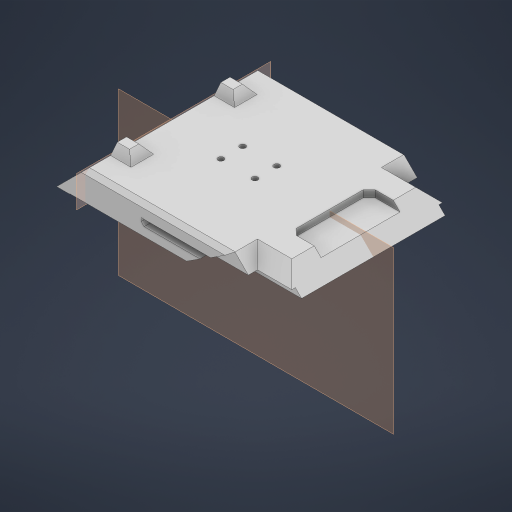
# Autodesk Inventor part: Head_Top
Saved by Autodesk Inventor 2024 (Build 280153000, 153)
## iProperties
Created: 2025-09-25
Part Number: Head_Top
Material: Generic
Document SubType Name: Modeling
Designer: kevin
Density: 1 g/cm^3
Appearance: Default
Author: kevin
Autodesk Inventor part; units mm, degrees
sketch "Sketch1" plane through (0, 0, 0) normal (0, 0, 1) x (1, 0, 0)
  line L0 (-49.5014, 88.2576) -> (-59.1834, 88.2576) projected
  line L1 (-18.2147, 2.3576) -> (-22.3392, 2.3576) projected
  arc A0 (-18.2147, 2.3576) -> (21.128, 5.3576) centre (0, 22.9604) ccw projected
  line L2 (103.9182, 5.3576) -> (21.128, 5.3576) projected
  line L3 (113.8557, 15.2951) -> (103.9182, 5.3576) projected
  line L4 (113.8557, 93.4201) -> (113.8557, 15.2951) projected
  line L5 (103.9182, 103.3576) -> (113.8557, 93.4201) projected
  line L6 (-46.9118, 103.3576) -> (103.9182, 103.3576) projected
  line L7 (-69.3743, 80.8951) -> (-46.9118, 103.3576) projected
  line L8 (-69.3743, 10.0256) -> (-69.3743, 80.8951) projected
  line L9 (-58.7063, -0.6424) -> (-69.3743, 10.0256) projected
  line L10 (-23.5178, -0.6424) -> (-58.7063, -0.6424) projected
  line L11 (-22.3392, 2.3576) -> (-23.5178, -0.6424) projected
  line L12 (-40.6109, 71.1084) -> (-33.5378, 60.1538) projected
  line L13 (-33.5378, 60.1538) -> (-15.7647, 71.6293) projected
  line L14 (-15.7647, 71.6293) -> (-15.7647, 88.2576) projected
  line L15 (-15.7647, 88.2576) -> (35.7434, 88.2576) projected
  line L16 (35.7434, 88.2576) -> (-58.3243, 27.521) projected
  line L17 (-58.3243, 27.521) -> (-58.3243, 44.1499) projected
  line L18 (-58.3243, 44.1499) -> (-49.3014, 49.9757) projected
  line L19 (-49.3014, 49.9757) -> (-49.3014, 71.1084) projected
  line L20 (-49.3014, 71.1084) -> (-40.6109, 71.1084) projected
  line L21 (3.2088, 99.2576) -> (52.78, 99.2576) projected
  line L22 (52.78, 99.2576) -> (46.5848, 95.2576) projected
  line L23 (46.5848, 95.2576) -> (5.2088, 95.2576) projected
  line L24 (3.2088, 97.2576) -> (5.2088, 95.2576) projected
  line L25 (3.2088, 97.2576) -> (3.2088, 99.2576) projected
  circle A1 centre (63.0077, 89.876) radius 2.1 projected
  line L26 (67.5987, 77.171) -> (76.5778, 68.1919) projected
  line L27 (76.5778, 68.1919) -> (76.5778, 21.8886) projected
  line L28 (76.5778, 21.8886) -> (68.2692, 13.58) projected
  line L29 (68.2692, 13.58) -> (19.2393, 13.58) projected
  line L30 (19.2393, 13.58) -> (11.6235, 21.1957) projected
  line L31 (11.6235, 21.1957) -> (67.5987, 77.171) projected
  line L32 (-59.1834, 88.2576) -> (-67.3743, 80.0667) projected
  line L33 (-59.1834, 88.2576) -> (-38.0834, 109.3576)
  line L34 (-46.9118, 103.3576) -> (103.9182, 103.3576) projected
  line L35 (68.9757, 109.3576) -> (117.3307, 109.3576) projected
  line L36 (68.9757, 109.3576) -> (-38.0834, 109.3576)
  line L37 (53.7977, 99.5576) -> (2.9088, 99.5576)
  line L38 (2.9088, 99.5576) -> (2.9088, 97.1333)
  line L39 (2.9088, 97.1333) -> (5.0845, 94.9576)
  line L40 (5.0845, 94.9576) -> (46.6733, 94.9576)
  line L41 (46.6733, 94.9576) -> (53.7977, 99.5576)
  line L42 (36.7611, 88.5576) -> (-16.0647, 88.5576)
  line L43 (-16.0647, 88.5576) -> (-16.0647, 71.7927)
  line L44 (-16.0647, 71.7927) -> (-33.4485, 60.5685)
  line L45 (-33.4485, 60.5685) -> (-40.4475, 71.4084)
  line L46 (-40.4475, 71.4084) -> (-49.6014, 71.4084)
  line L47 (-49.6014, 71.4084) -> (-49.6014, 50.1391)
  line L48 (-49.6014, 50.1391) -> (-58.6243, 44.3133)
  line L49 (-58.6243, 44.3133) -> (-58.6243, 26.9702)
  line L50 (-58.6243, 26.9702) -> (36.7611, 88.5576)
  line L51 (-16.0647, 88.5576) -> (-49.5014, 88.5576)
  line L52 (-49.5014, 88.5576) -> (-49.5014, 88.2576)
  line L53 (-56.6516, 28.2439) -> (64.3294, 106.3576) projected
  line L54 (-56.8143, 28.4959) -> (68.4226, 109.3576)
  line L55 (68.9757, 109.3576) -> (64.3294, 106.3576)
  point P0 (0, 0)
  point P1 (36.208, 88.5576)
  point P2 (46.1202, 94.9576)
  point P3 (53.2446, 99.5576)
  dimension "d0" = 0.3
  dimension "d1" = 0.3
  dimension "d2" = 0.3
  constraints: 40 end point, 2 horizontal, 1 parallel, 1 perpendicular, 1 point on line, 15 other
  measures "d0" distance between parallel lines of L21 L37
  measures "d1" distance between parallel lines of L15 L42
  measures "d2" distance between parallel lines of L53 L54
ref_plane "Work Plane1" through (-15.7647, 88.2576, 9.8) normal (0, 0.7071068, -0.7071068) x (0, 0.7071068, 0.7071068)
extrude "Extrusion1" add sketch "Sketch1" against normal up to surface contours L0 L33 L6 L54 L37 L38 L39 L40 L42 L51 L52 | L33 L36 L54 L6 | L54 L36 L55 L53 L6 | L6 L53 L37 L54 surface through (-15.7647, 88.2576, 9.8) normal (0, 0.7071068, -0.7071068)
ref_plane "Work Plane2" through (0, 0, 64.8) normal (0, 0, 1) x (1, 0, 0)
sketch "Sketch2" plane through (0, 0, 64.8) normal (0, 0, 1) x (1, 0, 0)
  line L0 (119.8557, 83.6682) -> (110.6663, 92.8576) projected
  line L1 (99.1663, 104.3576) -> (94.1663, 109.3576) projected
  line L2 (68.9757, 109.3576) -> (-38.0834, 109.3576) projected
  line L3 (-59.1834, 88.2576) -> (-49.5014, 88.2576) projected
  line L4 (-38.0834, 109.3576) -> (-59.1834, 88.2576) projected
  line L5 (68.9757, 109.3576) -> (94.1663, 109.3576) projected
  line L6 (-56.6516, 28.2439) -> (64.3294, 106.3576) projected
  line L7 (-56.6516, 28.2439) -> (64.3294, 106.3576) projected
  line L8 (53.7977, 99.5576) -> (68.9757, 109.3576) projected
  line L9 (-49.5014, 88.2576) -> (-49.5014, 88.5576) projected
  line L10 (-49.5014, 88.5576) -> (36.208, 88.5576) projected
  line L11 (46.1202, 94.9576) -> (5.0845, 94.9576) projected
  line L12 (46.1202, 94.9576) -> (46.6733, 94.9576)
  line L13 (5.0845, 94.9576) -> (-36.1716, 94.9576)
  line L14 (-36.1716, 94.9576) -> (-42.5716, 88.5576)
  point P0 (0, 0)
  dimension "d5" = 135
  constraints: 6 end point, 3 point on line, 1 horizontal
  measures "d5" angle of L13 L14
extrude "Extrusion2" add sketch "Sketch2" against normal up to surface surface through (4.8962, 98.8076, 20.35) normal (0, 0.7071068, -0.7071068)
sketch "Sketch3" plane through (0, 0, 64.8) normal (0, 0, 1) x (1, 0, 0)
  line L0 (119.8557, 83.6682) -> (110.6663, 92.8576) projected
  line L1 (99.1663, 104.3576) -> (94.1663, 109.3576) projected
  line L2 (68.9757, 109.3576) -> (94.1663, 109.3576) projected
  line L3 (99.1663, 104.3576) -> (112.3307, 104.3576) projected
  line L4 (110.6663, 92.8576) -> (99.1663, 104.3576)
  line L5 (-36.1716, 94.9576) -> (46.6733, 94.9576) projected
  line L6 (46.6733, 94.9576) -> (108.5663, 94.9576)
  line L7 (46.6733, 94.9576) -> (68.9757, 109.3576) projected
  line L8 (68.9757, 109.3576) -> (85.4757, 92.8576) projected
  line L9 (68.9757, 109.3576) -> (83.3757, 94.9576)
  line L10 (108.5663, 94.9576) -> (94.1663, 109.3576)
  line L11 (68.9757, 109.3576) -> (94.1663, 109.3576)
  point P0 (0, 0)
  constraints: 10 end point, 3 point on line, 2 collinear, 1 horizontal
ref_plane "Work Plane3" through (-8.0243, 5.3576, 2.8) normal (0, 0, 1) x (1, 0, 0)
extrude "Extrusion3" add sketch "Sketch3" against normal up to surface (62 mm away) contours L8 L6 L7
sketch "Sketch4" plane through (0, 0, 64.8) normal (0, 0, 1) x (1, 0, 0)
  line L0 (94.1663, 109.3576) -> (110.6663, 92.8576) projected
  line L1 (68.9757, 109.3576) -> (117.3307, 109.3576) projected
  line L2 (68.9757, 109.3576) -> (85.4757, 92.8576) projected
  line L3 (46.6733, 94.9576) -> (108.5663, 94.9576) projected
  point P0 (0, 0)
  point P1 (83.3757, 94.9576)
ref_plane "Work Plane4" through (68.9757, 92.8576, 2.8) normal (0, -0.7071068, 0.7071068) x (1, 0, 0)
extrude "Extrusion4" add sketch "Sketch4" against normal up to surface surface through (68.9757, 92.8576, 2.8) normal (0, -0.7071068, 0.7071068)
ref_plane "Work Plane5" through (7.9088, 97.1333, 0) normal (1, 0, 0) x (0, 0, -1)
sketch "Sketch6" plane through (7.9088, 97.1333, 0) normal (1, 0, 0) x (0, 0, -1)
  line L0 (0, -2.1757) -> (-16.5, -2.1757) projected
  line L1 (0.2, 0.1243) -> (0.2, -1.8757) projected
  line L2 (0.2, 0.1243) -> (0.2, 2.1243) projected
  line L3 (0, 2.4243) -> (-21.1, 2.4243) projected
  line L4 (-16.5, -2.1757) -> (-18.6757, 0) projected
  line L5 (-18.6757, 0) -> (-21.1, 2.4243) projected
  line L6 (0.2, 2.1243) -> (0.2, 2.4243)
  line L7 (0.2, 2.4243) -> (0, 2.4243)
  line L8 (0.2, -1.8757) -> (0, -2.1757)
  line L9 (-11.8, -25.504) -> (-11.8, -6.8757) projected
  line L10 (-12.1, -25.504) -> (-12.1, 2.4243)
  point P0 (0, -97.1333)
  point P1 (-12.1, -2.1757)
  dimension "d13" = 0.3
  constraints: 8 end point, 1 collinear, 1 parallel, 1 point on line, 1 vertical
  measures "d13" distance between parallel lines of L9 L10
extrude "Extrusion5" cut sketch "Sketch6" along normal blind 163.5125 contours L0 L10 L3 L7 L6 L2 L1 L8
chamfer "Chamfer1" distance 3 angle 45 1 edges at (15.4462, 109.3576, 0)
sketch "Sketch8" plane through (0, 0, 64.8) normal (0, 0, 1) x (1, 0, 0)
  line L0 (99.1663, 104.3576) -> (94.1663, 109.3576) projected
  line L1 (94.1663, 109.3576) -> (-38.0834, 109.3576) projected
  line L2 (99.1663, 104.3576) -> (76.5047, 104.3576)
  line L3 (76.5047, 104.3576) -> (71.5047, 109.3576)
  line L4 (108.5663, 94.9576) -> (94.1663, 109.3576) projected
  line L5 (76.5047, 104.3576) -> (76.5047, 109.3576)
  point P0 (0, 0)
  constraints: 6 end point, 2 point on line, 1 horizontal, 1 parallel, 1 perpendicular
ref_plane "Work Plane6" through (94.1663, 34.1725, 35.8) normal (0, 0, 1) x (1, 0, 0)
extrude "Extrusion6" cut sketch "Sketch8" against normal up to surface (29 mm away) contours L2 L5 L1 L0
mirror "Mirror2" about plane through (0, 0, 64.8) normal (0, 0, 1) of "Extrusion1", "Extrusion2", "Extrusion3", "Extrusion4", "Extrusion5", "Chamfer1", "Extrusion6"
sketch "Sketch10" plane through (-49.5014, 88.5576, 0) normal (0, -1, 0) x (1, 0, 0)
  line L0 (0, 129.6) -> (0, 0) projected
  circle A0 centre (5.406, 102.8115) radius 2.1
  circle A1 centre (5.406, 102.8115) radius 4.6
  line L1 (-43.2319, 64.8) -> (191.6177, 64.8) construction
  circle A2 centre (5.406, 102.8115) radius 5.1
  circle A3 centre (5.406, 26.7885) radius 2.1
  circle A4 centre (5.406, 26.7885) radius 4.6
  circle A5 centre (5.406, 26.7885) radius 5.1
  point P0 (49.5014, 0)
  dimension "d23" = 4.2
  dimension "d24" = 2.5
  dimension "d25" = 0.5
  constraints: 6 centre point, 1 symmetric about line, 3 other
  measures "d23" diameter of A0
  measures "d24" radial gap between concentric circles of A0 A1
  measures "d25" radial gap between concentric circles of A1 A2
extrude "Extrusion7" cut sketch "Sketch10" against normal blind 6 contours A0 | A1 | A2 | A3 | A4 | A5
sketch "Sketch11" plane through (-44.0955, 94.5576, 102.8115) normal (0, -1, 0) x (1, 0, 0)
  circle A0 centre (0, -76.023) radius 5.1 projected
  circle A1 centre (0, 0) radius 5.1 projected
  circle A2 centre (0, 0) radius 2.6
  circle A3 centre (0, -76.023) radius 2.6
  point P0 (44.0955, -102.8115)
  dimension "d28" = 5.2
  dimension "d29" = 5.2
  constraints: 2 centre point, 2 coincident
  measures "d28" diameter of A2
  measures "d29" diameter of A3
extrude "Extrusion8" cut sketch "Sketch11" against normal blind 31.4 contours A2 | A3
sketch "Sketch13" plane through (2.9088, 97.1333, 129.6) normal (1, 0, 0) x (0, 0, -1)
  line L0 (12.1, -2.1757) -> (12.1, 2.4243) projected
  line L1 (12.1, 2.4243) -> (21.1, 2.4243) projected
  line L2 (16.5, -2.1757) -> (21.1, 2.4243) projected
  line L3 (16.5, -2.1757) -> (12.1, -2.1757) projected
  line L4 (117.5, 2.4243) -> (117.5, -2.1757) projected
  line L5 (113.1, -2.1757) -> (117.5, -2.1757) projected
  line L6 (113.1, -2.1757) -> (108.5, 2.4243) projected
  line L7 (117.5, 2.4243) -> (108.5, 2.4243) projected
  point P0 (129.6, -97.1333)
extrude "Extrusion9" add sketch "Sketch13" along normal blind 53.625
sketch "Sketch14" plane through (76.5047, 104.3576, 35.8) normal (0, 1, 0) x (1, 0, 0)
  line L0 (22.6616, 0) -> (0, 0) projected
  line L1 (0, 0) -> (0, -58) projected
  line L2 (22.6616, -58) -> (0, -58) projected
  line L3 (22.6616, 0) -> (22.6616, -58) projected
  line L4 (0, -4.5253) -> (4.5253, 0)
  line L5 (0, 0) -> (17.6616, 0) projected
  line L6 (65.6116, -29) -> (-169.238, -29) construction
  line L7 (0, -53.4747) -> (4.5253, -58)
  point P0 (-76.5047, 35.8)
  point P1 (4.5253, -58)
  point P2 (0, -53.4747)
  point P3 (4.5253, 0)
  dimension "d34" = 45
  constraints: 4 end point, 2 point on line, 2 symmetric about line
  measures "d34" angle of L0 L4
extrude "Extrusion10" add sketch "Sketch14" along normal up to surface (5 mm away) contours L4 L1 L0 | L2 L1 L7
fillet "Fillet1" radius 1 6 edges at (-49.1955, 88.5576, 102.8115) (-39.9856, 91.1436, 99.7917) (-39.9856, 91.1436, 105.8313) (-49.1955, 88.5576, 26.7885) (-39.9856, 91.1436, 23.7687) (-39.9856, 91.1436, 29.8083)
sketch "Sketch15" plane through (68.9757, 109.3576, 19.3) normal (0, 1, 0) x (1, 0, 0)
  line L0 (7.529, -69.9747) -> (7.529, -21.0253) projected
  line L1 (12.0543, -16.5) -> (7.529, -21.0253) projected
  line L2 (12.0543, -16.5) -> (25.1906, -16.5) projected
  line L3 (25.1906, -16.5) -> (25.1906, 0) projected
  line L4 (0, 0) -> (25.1906, 0) projected
  line L5 (0, 0) -> (0, 16.3) projected
  line L6 (-107.0591, 16.3) -> (0, 16.3) projected
  line L7 (-107.0591, -107.3) -> (-107.0591, 16.3) projected
  line L8 (0, -107.3) -> (-107.0591, -107.3) projected
  line L9 (0, -91) -> (0, -107.3) projected
  line L10 (0, -91) -> (25.1906, -91) projected
  line L11 (25.1906, -74.5) -> (25.1906, -91) projected
  line L12 (25.1906, -74.5) -> (12.0543, -74.5) projected
  line L13 (7.529, -69.9747) -> (12.0543, -74.5) projected
  line L14 (7.529, -45.5) -> (-107.0591, -45.5) construction
  line L15 (7.529, -53.5) -> (-107.0591, -53.5) construction
  line L16 (7.529, -37.5) -> (-107.0591, -37.5) construction
  circle A0 centre (-39.3422, -53.5) radius 2.1
  circle A1 centre (-64.3422, -53.5) radius 2.1
  circle A2 centre (-64.3422, -37.5) radius 2.1
  circle A3 centre (-39.3422, -37.5) radius 2.1
  line L17 (-39.3422, -53.5) -> (-39.3422, -37.5) construction
  point P0 (-68.9757, 19.3)
  dimension "d38" = 8
  dimension "d39" = 8
  dimension "d40" = 4.2
  dimension "d41" = 4.2
  dimension "d42" = 4.2
  dimension "d43" = 4.2
  dimension "d44" = 25
  dimension "d45" = 25
  constraints: 8 end point, 4 centre point, 4 point on line, 2 midpoint, 2 parallel, 1 vertical
  measures "d38" distance between parallel lines of L14 L15
  measures "d39" distance between parallel lines of L14 L16
  measures "d40" diameter of A0
  measures "d41" diameter of A1
  measures "d42" diameter of A2
  measures "d43" diameter of A3
  measures "d44" distance of A1.centre L17.start
  measures "d45" distance of A2.centre L17.end
extrude "Extrusion11" cut sketch "Sketch15" against normal blind 25.4 contours A0 | A1 | A2 | A3
ref_plane "Work Plane7" through (-38.0834, 109.3576, 129.6) normal (1, 0, 0) x (0, 0, -1)
sketch "Sketch16" plane through (-38.0834, 109.3576, 129.6) normal (1, 0, 0) x (0, 0, -1)
  circle A0 centre (102.8115, -6.0121) radius 2.6 projected
  circle A1 centre (26.7885, -6.0121) radius 2.6 projected
  line L0 (102.8115, -3.4121) -> (102.8115, 3.5903) construction
  line L1 (26.7885, -3.4121) -> (26.7885, 2.586) construction
  line L2 (3, 0) -> (126.6, 0) projected
  line L3 (2.9538, 6) -> (126.5538, 6)
  line L4 (111.1084, 0) -> (106.2087, 6)
  line L5 (94.5147, 0) -> (99.4143, 6)
  line L6 (64.8, 0) -> (64.8, 3) construction
  line L7 (18.4916, 0) -> (23.3913, 6)
  line L8 (35.0853, 0) -> (30.1857, 6)
  point P0 (129.6, -109.3576)
  point P1 (23.3913, 6)
  point P2 (18.4916, 0)
  point P3 (35.0853, 0)
  point P4 (30.1857, 6)
  point P5 (99.4143, 6)
  point P6 (94.5147, 0)
  dimension "d49" = 6
  constraints: 16 end point, 6 symmetric about line, 3 vertical, 2 point on line, 2 vertical alignment, 1 midpoint, 1 parallel, 2 other
  measures "d49" distance between parallel lines of L2 L3
extrude "Extrusion12" add sketch "Sketch16" along normal blind 15 contours L7 L3 L8 L2 | L5 L3 L4 L2
chamfer "Chamfer2" distance 6 angle 45 2 edges at (-23.0834, 115.3576, 26.7885) (-23.0834, 115.3576, 102.8115)
equation "\"d39\" = d38"
equation "\"d45\" = d44"
body "Solid1"
